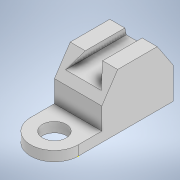
# Autodesk Inventor part: Ch4 Part 4
Saved by Autodesk Inventor 2020 (Build 240168000, 168)
## iProperties
Created: 2021-02-11
Part Number: Ch4 Part 4
Material: Generic
Document SubType Name: Modeling
Designer: austi
Density: 1 g/cm^3
Appearance: Default
Author: austi
Autodesk Inventor part; units mm, degrees
ref_plane "YZ Plane" through (0, 0, 0) normal (1, 0, 0) x (0, 1, 0)
ref_plane "XZ Plane" through (0, 0, 0) normal (0, 1, 0) x (-1, 0, 0)
ref_plane "XY Plane" through (0, 0, 0) normal (0, 0, 1) x (1, 0, 0)
sketch "Sketch1" plane through (0, 0, 0) normal (0, 1, 0) x (-1, 0, 0)
  arc A0 (38.1, 0) -> (-38.1, 0) centre (0, 0) ccw
  line L0 (38.1, 0) -> (38.1, -152.4)
  line L1 (-38.1, 0) -> (-38.1, -152.4)
  line L2 (0, -190.5) -> (0, 76.2) projected
  line L3 (53.34, 0) -> (-53.34, 0) projected
  line L4 (38.1, -152.4) -> (-38.1, -152.4)
  dimension "d0" = 76.2
  dimension "d1" = 152.4
  dimension "d2" = 152.4
  constraints: 6 end point, 2 point on circle, 2 point on line, 2 vertical, 1 centre point, 1 coincident, 1 tangent, 1 other
  measures "d0" diameter of A0
  measures "d1" distance of L0.start L0.end
  measures "d2" distance of L1.start L1.end
extrude "Extrusion1" add sketch "Sketch1" along normal blind 15.875
sketch "Sketch2" plane through (0, 15.875, 0) normal (0, 1, 0) x (1, 0, 0)
  point P0 (0, 0)
  point P1 (0, 0)
  constraints: 1 coincident
hole "Hole1" at (0, 15.875, 0) direction (0, -1, 0) diameter 38.1 depth 15.875 tip angle 118
sketch "Sketch4" plane through (38.1, 0, 0) normal (1, 0, 0) x (0, 0, -1)
  line L0 (152.4, 15.875) -> (0, 15.875) projected
  line L1 (152.4, 15.875) -> (152.4, 50.8)
  line L2 (152.4, 50.8) -> (152.4, 88.9)
  line L3 (152.4, 88.9) -> (38.1, 88.9)
  line L4 (38.1, 88.9) -> (38.1, 15.875)
  line L5 (152.4, 50.8) -> (127, 88.9)
  line L6 (38.1, 50.8) -> (63.5, 88.9)
  line L7 (46.5667, 63.5) -> (143.9333, 63.5)
  point P0 (0, 0)
  dimension "d15" = 114.3
  dimension "d16" = 50.8
  dimension "d17" = 88.9
  dimension "d18" = 25.4
  dimension "d19" = 25.4
  constraints: 14 end point, 7 point on line, 2 perpendicular, 1 equal length, 1 horizontal, 1 horizontal alignment, 1 vertical
  measures "d15" distance of L2.end L3.end
  measures "d16" vertical distance of L1.end point (0, 0)
  measures "d17" vertical distance of L2.end point (0, 0)
  measures "d18" distance of L2.end L5.end
  measures "d19" vertical distance of L3.end L7.start
extrude "Extrusion2" add sketch "Sketch4" against normal blind 76.2 contours L0 L4 L6 L7 L5 L1
shell "Shell1" thickness 4.7625 removed faces 1 at (0, 0, -107.95)
sketch "Sketch5" plane through (38.1, 0, 0) normal (1, 0, 0) x (0, 0, -1)
  point P0 (0, 0)
sketch "Sketch6" plane through (38.1, 0, 0) normal (1, 0, 0) x (0, 0, -1)
  line L0 (38.1, 50.8) -> (38.1, 15.875) projected
  line L1 (38.1, 50.8) -> (38.1, 88.9)
  line L2 (38.1, 88.9) -> (152.4, 88.9)
  line L3 (152.4, 0) -> (152.4, 50.8) projected
  line L4 (152.4, 88.9) -> (152.4, 50.8)
  line L5 (46.5667, 63.5) -> (38.1, 50.8) projected
  line L6 (46.5667, 63.5) -> (63.5, 88.9)
  line L7 (152.4, 50.8) -> (143.9333, 63.5) projected
  line L8 (143.9333, 63.5) -> (127, 88.9)
  line L9 (46.5667, 63.5) -> (143.9333, 63.5)
  line L10 (0, 0) -> (152.4, 0) projected
  dimension "d23" = 38.1
  constraints: 12 end point, 2 collinear, 2 perpendicular, 2 point on line, 1 parallel, 1 vertical
  measures "d23" distance of L0.start L1.end
extrude "Extrusion3" add sketch "Sketch6" against normal blind 76.2 contours L6 L2 L8 L9
sketch "Sketch8" plane through (38.1, 15.875, -38.1) normal (0, 0, 1) x (1, 0, 0)
  line L0 (-66.675, 47.625) -> (-9.525, 47.625)
  line L1 (0, 73.025) -> (-76.2, 73.025) projected
  line L2 (-66.675, 47.625) -> (-52.0103, 73.025)
  line L3 (-9.525, 47.625) -> (-24.1897, 73.025)
  line L4 (-52.0103, 73.025) -> (-24.1897, 73.025)
  point P0 (-38.1, -15.875)
  point P1 (-59.3427, 60.325)
  point P2 (-16.8573, 60.325)
  point P3 (-38.1, 73.025)
  point P4 (-38.1, 47.625)
  dimension "d31" = 57.15
  dimension "d32" = 25.4
  dimension "d33" = 60
  constraints: 8 end point, 4 midpoint, 3 point on line, 2 horizontal alignment, 1 equal length, 1 horizontal, 1 vertical alignment
  measures "d31" distance of L0.start L0.end
  measures "d32" distance from line of L1 L0.start
  measures "d33" angle of L0 L2
extrude "Extrusion4" cut sketch "Sketch8" against normal blind 107.95
body "Solid1"
